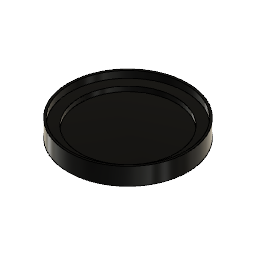
19) PLA Bath (Autodesk Fusion 360 design; units mm, degrees)
Autodesk Fusion 360 part; units mm, degrees
sketch "Sketch1" plane through (0, 0, 0) normal (0, 1, 0) x (1, 0, 0)
  line L0 (0, 11) -> (62, 11)
  line L1 (62, 11) -> (62, -7)
  line L2 (62, -7) -> (60, -7)
  line L3 (60, -7) -> (60, 0)
  line L4 (60, 0) -> (50, 0)
  line L5 (50, 0) -> (50, 5)
  line L6 (50, 5) -> (0, 5)
  line L7 (0, 5) -> (0, 11)
  line L8 (50, 0) -> (0, 0) construction
  line L9 (0, 0) -> (0, 5) construction
  dimension "d2" = 50
  dimension "d3" = 10
  dimension "d4" = 2
  dimension "d5" = 5
  dimension "d6" = 7
  dimension "d7" = 6
  constraint horizontal L0
  constraint perpendicular L0 L1
  constraint perpendicular L1 L2
  constraint perpendicular L2 L3
  constraint perpendicular L3 L4
  constraint perpendicular L4 L5
  constraint perpendicular L5 L6
  constraint perpendicular L6 L7
  constraint coincident L0.start L7.end
  constraint perpendicular L5 L8
  constraint perpendicular L8 L9
  constraint coincident L8.end L9.start
  measures "d2" distance of L5 L6.end
  measures "d3" distance of L3.end L4.end
  measures "d4" distance of L1.end L2.end
  measures "d5" distance of L4.end L5.end
  measures "d6" distance of L2.end L3.end
  measures "d7" distance of L0 L6
revolve "Revolve1" add sketch "Sketch1" angle 360 about axis through (0, 0, 0) along (0, 0, -1) makes body 1
sketch "Sketch1 (1)" plane through (0, 0, 0) normal (0, 1, 0) x (1, 0, 0)
  line L0 (-25, 8) -> (-25, 11)
  line L1 (-22, 8) -> (-25, 8)
  line L2 (-25, 11) -> (0, 11)
  line L3 (0, 11) -> (0, 8)
  line L4 (0, 8) -> (-22, 8)
  line L5 (0, 0) -> (0, 8)
  constraint perpendicular L0 L2
  constraint perpendicular L2 L3
  constraint coincident L1.start L4.end
  constraint horizontal L4
  constraint coincident L5.start origin
  constraint vertical L5
  constraint coincident L0.end L2.start
revolve "Revolve2" cut sketch "Sketch1 (1)" angle 360 about axis through (0, 0, 0) along (0, 0, -1) bodies 1
thread "Thread1" "ISO Metric profile 50.0 M50x2 M50x2 6H" major diameter 50.2623 minor diameter 48.0224 pitch 2 angle 60 modelled right hand crest width 0.5401 on face at (-24.9689, -1.2461, -9) crest through (-24.0112, 0, -8.5) on bodies 1
sketch "Sketch2" plane through (0, 0, 0) normal (0, 1, 0) x (1, 0, 0)
  line L0 (-25, 8) -> (-25, 11)
  line L1 (-25, 11) -> (0, 11)
  line L2 (-25, 11) -> (-23.5, 9.5)
  line L3 (-23.5, 9.5) -> (-23.5, 11)
  dimension "d130" = 45
  dimension "d131" = 1.5
  constraint coincident L0.end L1.start
  constraint coincident L1 L3.end
  constraint perpendicular L1 L3
  measures "d130" angle of L1 L2
  measures "d131" distance of L0.end L3.end
revolve "Revolve3" cut sketch "Sketch2" angle 360 about axis through (0, 0, -205.75) along (0, 0, 1) bodies 1
copy_body "Body->Comp1" bodies 1 removing the originals makes body 2 in component "100mm Bath"
sketch "Sketch1 (2)" plane through (0, 0, 0) normal (0, 1, 0) x (1, 0, 0) in component "40mm square bath"
  line L0 (-25, 11) -> (0, 11) construction
  line L1 (-25, 8) -> (-25, 11) construction
  line L2 (62, 11) -> (62, -7) construction
  line L3 (62, -7) -> (60, -7) construction
  line L4 (60, -7) -> (60, 0) construction
  line L5 (60, 0) -> (50, 0) construction
  line L6 (50, 0) -> (50, 5) construction
  line L7 (50, 5) -> (0, 5) construction
  line L8 (0, 11) -> (62, 11) construction
  line L9 (0, 11) -> (-25, 11)
  line L10 (-25, 11) -> (-25, 8)
  line L11 (-25, 8) -> (0, 8)
  line L12 (0, 8) -> (0, 11)
  line L13 (-25, 11) -> (-40, 11)
  line L14 (-40, 11) -> (-40, -7)
  line L15 (-40, -7) -> (-38, -7)
  line L16 (-38, -7) -> (-38, 0)
  line L17 (-38, 0) -> (-10, 0)
  line L18 (-10, 0) -> (-10, 5)
  line L19 (-10, 5) -> (0, 5)
  line L20 (0, 8) -> (0, 5)
  dimension "d205" = 40
  dimension "d206" = 2
  dimension "d208" = 10
  constraint horizontal L9
  constraint horizontal L11
  constraint vertical L12
  constraint coincident L1.start L10.end
  constraint coincident L0.end L8.start
  constraint coincident L0.start L1.end
  constraint perpendicular L13 L14
  constraint perpendicular L14 L15
  constraint perpendicular L15 L16
  constraint perpendicular L16 L17
  constraint perpendicular L17 L18
  constraint coincident L7.end L19.end
  constraint horizontal L19
  constraint collinear L5 L17
  constraint collinear L3 L15
  measures "d205" distance of L12 L14
  measures "d206" distance of L14.end L15.end
  measures "d208" distance of L18.end L7.end
revolve "Revolve1'" add sketch "Sketch1 (2)" angle 360 about axis through (0, 0, -8) along (0, 0, 1) separate body contours L10 L11 L13 L14 L15 L16 L17 L18 L19 L20 makes body 3 in component "40mm square bath"
sketch "Sketch2 (2)" plane through (0, 0, 0) normal (0, 0, 1) x (-1, 0, 0) in component "40mm square bath"
  circle A0 centre (0, 0) radius 10 construction
  circle A1 centre (0, 0) radius 38 construction
  line L0 (20, -20) -> (-20, -20)
  line L1 (-20, -20) -> (-20, 20)
  line L2 (-20, 20) -> (20, 20)
  line L3 (20, 20) -> (20, -20)
  line L4 (-20, -20) -> (20, 20) construction
  dimension "d210" = 40
  dimension "d211" = 40
  constraint horizontal L0
  constraint vertical L1
  constraint horizontal L2
  constraint vertical L3
  constraint midpoint A0.centre L4
  measures "d210" distance of L0.start L0.end
  measures "d211" distance of L0.start L2.end
extrude "Extrude1" cut sketch "Sketch2 (2)" against normal up to surface (5 mm away) bodies 3 in component "40mm square bath"
thread "Thread1'" "ISO Metric profile 50.0 M50x2 M50x2 6H" major diameter 50.2623 minor diameter 48.0224 pitch 2 angle 60 modelled right hand crest width 0.5401 on face at (-24.9689, 1.2461, -10) crest through (-24.0112, 0, -8.5) on bodies 3 in component "40mm square bath"
sketch "Sketch3" plane through (0, 0, 0) normal (0, 1, 0) x (1, 0, 0) in component "40mm square bath"
  line L0 (0, 11) -> (-25, 11)
  line L1 (-25, 11) -> (-23.5, 9.5)
  line L2 (-23.5, 9.5) -> (-23.5, 11)
  dimension "d220" = 1.5
  dimension "d221" = 45
  constraint coincident L0.end L1.start
  constraint coincident L0 L2.end
  constraint perpendicular L0 L2
  measures "d220" distance of L0.end L2.end
  measures "d221" angle of L0 L1
revolve "Revolve3'" cut sketch "Sketch3" angle 360 about axis through (0, 0, -205.75) along (0, 0, 1) bodies 3 in component "40mm square bath"
component "40mm square bath" placed x (1, 0, 0) y (0, 1, 0) z (0, 0, 1) at (0, 0, 0)
component "100mm Bath" placed x (1, 0, 0) y (0, 1, 0) z (0, 0, 1) at (0, 0, 0)
